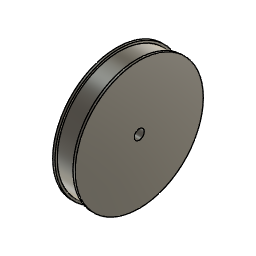
wheel (Autodesk Fusion 360 design; units mm, degrees)
Autodesk Fusion 360 part; units mm, degrees
sketch "Sketch6" plane through (0, 0, 0) normal (1, 0, 0) x (0, 1, 0)
  circle A0 centre (0, 0) radius 27.5
  circle A1 centre (0, 0) radius 22.5
  dimension "d30" = 55
  dimension "d31" = 45
  constraint coincident A0.centre A1.centre
  constraint concentric A0 A1
  measures "d30" diameter of A0
  measures "d31" diameter of A1
extrude "Extrude11" add sketch "Sketch6" along normal blind 10 makes body 1
sketch "Sketch7" plane through (10, 0, 0) normal (1, 0, 0) x (0, 1, 0)
  circle A0 centre (0, 0) radius 22.5
  circle A1 centre (0, 0) radius 27.5
  circle A2 centre (0, 0) radius 27.5
  line L0 (0, 0) -> (0, 27.5)
  line L1 (0, 27.5) -> (-2, 27.5)
  line L2 (-2, 27.5) -> (2, 27.5)
  line L3 (0, 0) -> (3, 0)
  line L4 (3, 0) -> (-3, 0)
  line L5 (-3, 0) -> (-2, 27.5)
  line L6 (3, 0) -> (2, 27.5)
  dimension "d34" = 2
  dimension "d35" = 4
  dimension "d36" = 3
  constraint concentric A0 A2
  constraint coincident A0.centre A1.centre
  constraint coincident A2 L0.end
  constraint vertical L0
  constraint perpendicular L0 L1
  constraint perpendicular L0 L2
  constraint perpendicular L0 L3
  constraint perpendicular L0 L4
  measures "d34" distance of L0.end L1.end
  measures "d35" distance of L1.end L2.end
  measures "d36" distance of A0.centre L3.end
extrude "Extrude12" add sketch "Sketch7" along normal blind 2 separate body contours A0 L0 L3 L4 L6 | A0 L0 L4 L5 makes body 2
pattern_circular "C-Pattern2" count 10 over 360 about axis through (10, 0, 0) along (-1, 0, 0) of bodies 2 makes body 3 at (10, 2.9891, 7.055) makes body 4 at (10, 6.565, 3.9506) makes body 5 at (10, 7.6333, -0.6627) makes body 6 at (10, 5.786, -5.0229) makes body 7 at (10, 1.7286, -7.4645) makes body 8 at (10, -2.9891, -7.055) makes body 9 at (10, -6.565, -3.9506) makes body 10 at (10, -7.6333, 0.6627) makes body 11 at (10, -5.786, 5.0229)
combine "Combine2" operation add target body 2 tool bodies 6 7 4 5 3 8 9 10 11
extrude "Extrude13" add 1 faces at (10, 1.4552, -1.0572) along direction (-1, 0, 0) blind 6 on bodies 2 bodies 1 2
extrude "Extrude14" cut 1 faces at (12, 1.4552, -1.0572) along direction (-1, 0, 0) blind 2 on bodies 1 bodies 1
sketch "Sketch8" plane through (10, 0, 0) normal (1, 0, 0) x (0, 1, 0)
  arc A0 (2.1857, -22.3936) -> (11.3944, -19.4015) centre (0, 0) ccw
  line L0 (2.1857, -22.3936) -> (2.698, -8.3037)
  line L1 (2.698, -8.3037) -> (11.3944, -19.4015)
  line L2 (14.9309, -16.8321) -> (7.0636, -5.132)
  line L3 (7.0636, -5.132) -> (20.6222, -8.9987)
  arc A1 (14.9309, -16.8321) -> (20.6222, -8.9987) centre (0, 0) ccw
  arc A2 (-11.3944, -19.4015) -> (-2.1857, -22.3936) centre (0, 0) ccw
  line L4 (-11.3944, -19.4015) -> (-2.698, -8.3037)
  line L5 (-2.698, -8.3037) -> (-2.1857, -22.3936)
  line L6 (21.973, -4.8413) -> (8.7311, 0)
  line L7 (8.7311, 0) -> (21.973, 4.8413)
  arc A3 (21.973, -4.8413) -> (21.973, 4.8413) centre (0, 0) ccw
  arc A4 (-20.6222, -8.9987) -> (-14.9309, -16.8321) centre (0, 0) ccw
  line L8 (-20.6222, -8.9987) -> (-7.0636, -5.132)
  line L9 (-7.0636, -5.132) -> (-14.9309, -16.8321)
  line L10 (20.6222, 8.9987) -> (7.0636, 5.132)
  line L11 (7.0636, 5.132) -> (14.9309, 16.8321)
  arc A5 (20.6222, 8.9987) -> (14.9309, 16.8321) centre (0, 0) ccw
  arc A6 (-21.973, 4.8413) -> (-21.973, -4.8413) centre (0, 0) ccw
  line L12 (-21.973, 4.8413) -> (-8.7311, 0)
  line L13 (-8.7311, 0) -> (-21.973, -4.8413)
  line L14 (11.3944, 19.4015) -> (2.698, 8.3037)
  line L15 (2.698, 8.3037) -> (2.1857, 22.3936)
  arc A7 (11.3944, 19.4015) -> (2.1857, 22.3936) centre (0, 0) ccw
  arc A8 (-14.9309, 16.8321) -> (-20.6222, 8.9987) centre (0, 0) ccw
  line L16 (-14.9309, 16.8321) -> (-7.0636, 5.132)
  line L17 (-7.0636, 5.132) -> (-20.6222, 8.9987)
  line L18 (-2.1857, 22.3936) -> (-2.698, 8.3037)
  line L19 (-2.698, 8.3037) -> (-11.3944, 19.4015)
  arc A9 (-2.1857, 22.3936) -> (-11.3944, 19.4015) centre (0, 0) ccw
  circle A10 centre (0, 0) radius 27.5
  circle A11 centre (0, 0) radius 27.5
  constraint concentric A0 A11
extrude "Extrude15" add sketch "Sketch8" against normal blind 3 contours A0 L0 L1 | L2 L3 A1 | A2 L4 L5 | L6 L7 A3 | A4 L8 L9 | L10 L11 A5 | A6 L12 L13 | L14 L15 A7 | A8 L16 L17 | L18 L19 A9 bodies 1
extrude "Extrude16" add 1 faces at (4, 1.4552, -1.0572) along direction (-1, 0, 0) blind 2 on bodies 1 bodies 1
sketch "Sketch9" plane through (2, 0, 0) normal (-1, 0, 0) x (0, -1, 0)
  line L0 (7.0636, 5.132) -> (14.9309, 16.8321)
  arc A0 (14.9309, 16.8321) -> (11.3944, 19.4015) centre (0, 0) ccw
  line L1 (11.3944, 19.4015) -> (2.698, 8.3037)
  line L2 (2.698, 8.3037) -> (2.1857, 22.3936)
  arc A1 (2.1857, 22.3936) -> (-2.1857, 22.3936) centre (0, 0) ccw
  line L3 (-2.1857, 22.3936) -> (-2.698, 8.3037)
  line L4 (-2.698, 8.3037) -> (-11.3944, 19.4015)
  arc A2 (-11.3944, 19.4015) -> (-14.9309, 16.8321) centre (0, 0) ccw
  line L5 (-14.9309, 16.8321) -> (-7.0636, 5.132)
  line L6 (-7.0636, 5.132) -> (-20.6222, 8.9987)
  arc A3 (-20.6222, 8.9987) -> (-21.973, 4.8413) centre (0, 0) ccw
  line L7 (-21.973, 4.8413) -> (-8.7311, 0)
  line L8 (-8.7311, 0) -> (-21.973, -4.8413)
  arc A4 (-21.973, -4.8413) -> (-20.6222, -8.9987) centre (0, 0) ccw
  line L9 (-20.6222, -8.9987) -> (-7.0636, -5.132)
  line L10 (-7.0636, -5.132) -> (-14.9309, -16.8321)
  arc A5 (-14.9309, -16.8321) -> (-11.3944, -19.4015) centre (0, 0) ccw
  line L11 (-11.3944, -19.4015) -> (-2.698, -8.3037)
  line L12 (-2.698, -8.3037) -> (-2.1857, -22.3936)
  arc A6 (-2.1857, -22.3936) -> (2.1857, -22.3936) centre (0, 0) ccw
  line L13 (2.1857, -22.3936) -> (2.698, -8.3037)
  line L14 (2.698, -8.3037) -> (11.3944, -19.4015)
  arc A7 (11.3944, -19.4015) -> (14.9309, -16.8321) centre (0, 0) ccw
  line L15 (14.9309, -16.8321) -> (7.0636, -5.132)
  line L16 (7.0636, -5.132) -> (20.6222, -8.9987)
  arc A8 (20.6222, -8.9987) -> (21.973, -4.8413) centre (0, 0) ccw
  line L17 (21.973, -4.8413) -> (8.7311, 0)
  line L18 (8.7311, 0) -> (21.973, 4.8413)
  arc A9 (21.973, 4.8413) -> (20.6222, 8.9987) centre (0, 0) ccw
  line L19 (20.6222, 8.9987) -> (7.0636, 5.132)
  circle A10 centre (0, 0) radius 2.75
  dimension "d49" = 5.5
  constraint coincident A0.centre A1.centre
  measures "d49" diameter of A10
extrude "Extrude17" cut sketch "Sketch9" against normal blind 10 contours A10 bodies 1
fillet "Fillet2" radius 2.5 1 edges at (2, 2.5639, 0.9944) on bodies 1
sketch "Sketch10" plane through (0, 0, 0) normal (-1, 0, 0) x (0, -1, 0)
  circle A0 centre (0, 0) radius 22.5
  circle A1 centre (0, 0) radius 27.5
  circle A2 centre (0, 0) radius 28.5
  dimension "d54" = 57
  constraint coincident A0.centre A1.centre
  measures "d54" diameter of A2
extrude "Extrude18" add sketch "Sketch10" against normal blind 2 contours A2 bodies 1
sketch "Sketch11" plane through (10, 0, 0) normal (1, 0, 0) x (0, 1, 0)
  circle A0 centre (0, 0) radius 2.75
  circle A1 centre (0, 0) radius 27.5
  circle A2 centre (0, 0) radius 28.5
  dimension "d57" = 57
  constraint concentric A0 A2
  measures "d57" diameter of A2
extrude "Extrude19" add sketch "Sketch11" against normal blind 2 contours A2 bodies 1
extrude "Extrude20" cut 1 faces at (2, -27.9582, -2.7821) along direction (-1, 0, 0) blind 1 on bodies 1 bodies 1
extrude "Extrude21" cut 1 faces at (8, 27.9582, -2.7821) along direction (1, 0, 0) blind 1 on bodies 1 bodies 1
delete_face "DeleteFace1" 1 faces at (2.0024, -4.7373, -1.9969) on bodies 1
sketch "Sketch12" plane through (2, 0, 0) normal (-1, 0, 0) x (0, -1, 0)
  line L0 (7.0636, 5.132) -> (14.9309, 16.8321)
  arc A0 (14.9309, 16.8321) -> (11.3944, 19.4015) centre (0, 0) ccw
  line L1 (11.3944, 19.4015) -> (2.698, 8.3037)
  line L2 (2.698, 8.3037) -> (2.1857, 22.3936)
  arc A1 (2.1857, 22.3936) -> (-2.1857, 22.3936) centre (0, 0) ccw
  line L3 (-2.1857, 22.3936) -> (-2.698, 8.3037)
  line L4 (-2.698, 8.3037) -> (-11.3944, 19.4015)
  arc A2 (-11.3944, 19.4015) -> (-14.9309, 16.8321) centre (0, 0) ccw
  line L5 (-14.9309, 16.8321) -> (-7.0636, 5.132)
  line L6 (-7.0636, 5.132) -> (-20.6222, 8.9987)
  arc A3 (-20.6222, 8.9987) -> (-21.973, 4.8413) centre (0, 0) ccw
  line L7 (-21.973, 4.8413) -> (-8.7311, 0)
  line L8 (-8.7311, 0) -> (-21.973, -4.8413)
  arc A4 (-21.973, -4.8413) -> (-20.6222, -8.9987) centre (0, 0) ccw
  line L9 (-20.6222, -8.9987) -> (-7.0636, -5.132)
  line L10 (-7.0636, -5.132) -> (-14.9309, -16.8321)
  arc A5 (-14.9309, -16.8321) -> (-11.3944, -19.4015) centre (0, 0) ccw
  line L11 (-11.3944, -19.4015) -> (-2.698, -8.3037)
  line L12 (-2.698, -8.3037) -> (-2.1857, -22.3936)
  arc A6 (-2.1857, -22.3936) -> (2.1857, -22.3936) centre (0, 0) ccw
  line L13 (2.1857, -22.3936) -> (2.698, -8.3037)
  line L14 (2.698, -8.3037) -> (11.3944, -19.4015)
  arc A7 (11.3944, -19.4015) -> (14.9309, -16.8321) centre (0, 0) ccw
  line L15 (14.9309, -16.8321) -> (7.0636, -5.132)
  line L16 (7.0636, -5.132) -> (20.6222, -8.9987)
  arc A8 (20.6222, -8.9987) -> (21.973, -4.8413) centre (0, 0) ccw
  line L17 (21.973, -4.8413) -> (8.7311, 0)
  line L18 (8.7311, 0) -> (21.973, 4.8413)
  arc A9 (21.973, 4.8413) -> (20.6222, 8.9987) centre (0, 0) ccw
  line L19 (20.6222, 8.9987) -> (7.0636, 5.132)
  circle A10 centre (0, 0) radius 2.75
  circle A11 centre (0, 0) radius 2.55
  dimension "d64" = 5.1
  constraint coincident A0.centre A1.centre
  measures "d64" diameter of A11
extrude "Extrude22" add sketch "Sketch12" against normal blind 8 contours A10 bodies 1
scale "Scale1" factor 1.14 about (1, 27.5, 0) bodies 1
sketch "Sketch13" plane through (2.14, 0, 0) normal (-1, 0, 0) x (0, -1, 0)
  circle A0 centre (3.85, 0) radius 2.907
  line L0 (11.9025, 5.8505) -> (20.8712, 19.1886)
  arc A1 (20.8712, 19.1886) -> (16.8396, 22.1177) centre (3.85, 0) ccw
  line L1 (16.8396, 22.1177) -> (6.9258, 9.4663)
  line L2 (6.9258, 9.4663) -> (6.3417, 25.5287)
  arc A2 (6.3417, 25.5287) -> (1.3583, 25.5287) centre (3.85, 0) ccw
  line L3 (1.3583, 25.5287) -> (0.7742, 9.4663)
  line L4 (0.7742, 9.4663) -> (-9.1396, 22.1177)
  arc A3 (-9.1396, 22.1177) -> (-13.1712, 19.1886) centre (3.85, 0) ccw
  line L5 (-13.1712, 19.1886) -> (-4.2025, 5.8505)
  line L6 (-4.2025, 5.8505) -> (-19.6593, 10.2585)
  arc A4 (-19.6593, 10.2585) -> (-21.1992, 5.5191) centre (3.85, 0) ccw
  line L7 (-21.1992, 5.5191) -> (-6.1034, 0)
  line L8 (-6.1034, 0) -> (-21.1992, -5.5191)
  arc A5 (-21.1992, -5.5191) -> (-19.6593, -10.2585) centre (3.85, 0) ccw
  line L9 (-19.6593, -10.2585) -> (-4.2025, -5.8505)
  line L10 (-4.2025, -5.8505) -> (-13.1712, -19.1886)
  arc A6 (-13.1712, -19.1886) -> (-9.1396, -22.1177) centre (3.85, 0) ccw
  line L11 (-9.1396, -22.1177) -> (0.7742, -9.4663)
  line L12 (0.7742, -9.4663) -> (1.3583, -25.5287)
  arc A7 (1.3583, -25.5287) -> (6.3417, -25.5287) centre (3.85, 0) ccw
  line L13 (6.3417, -25.5287) -> (6.9258, -9.4663)
  line L14 (6.9258, -9.4663) -> (16.8396, -22.1177)
  arc A8 (16.8396, -22.1177) -> (20.8712, -19.1886) centre (3.85, 0) ccw
  line L15 (20.8712, -19.1886) -> (11.9025, -5.8505)
  line L16 (11.9025, -5.8505) -> (27.3593, -10.2585)
  arc A9 (27.3593, -10.2585) -> (28.8992, -5.5191) centre (3.85, 0) ccw
  line L17 (28.8992, -5.5191) -> (13.8034, 0)
  line L18 (13.8034, 0) -> (28.8992, 5.5191)
  arc A10 (28.8992, 5.5191) -> (27.3593, 10.2585) centre (3.85, 0) ccw
  line L19 (27.3593, 10.2585) -> (11.9025, 5.8505)
  circle A11 centre (3.85, 0) radius 2.55
  dimension "d68" = 5.1
  constraint concentric A0 A11
  measures "d68" diameter of A11
extrude "Extrude23" add sketch "Sketch13" against normal blind 9.12 contours A0 bodies 1
equation "d55 = 2 mm - 4 mm"
equation "d69 = ( -8 * 1.14 ) * 1 mm"
